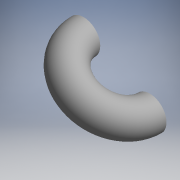
# Autodesk Inventor part: Half Off-Axis Donut Revolve Demo
Saved by Autodesk Inventor 2019 (Build 230136000, 136)
## iProperties
Part Number: Half Off-Axis Donut Revolve Demo
Material: Generic
Document SubType Name: Modeling
Designer: oriani
Appearance: Default
Author: oriani
Autodesk Inventor part; units mm, degrees
ref_plane "YZ Plane" through (0, 0, 0) normal (1, 0, 0) x (0, 1, 0)
ref_plane "XZ Plane" through (0, 0, 0) normal (0, 1, 0) x (-1, 0, 0)
ref_plane "XY Plane" through (0, 0, 0) normal (0, 0, 1) x (1, 0, 0)
sketch "Sketch1" plane through (0, 0, 0) normal (0, 0, 1) x (1, 0, 0)
  circle A0 centre (0, 25.4) radius 5.08
  line L0 (0, 0) -> (6.35, 12.7)
  dimension "d0" = 0
  constraints: 2 end point, 1 centre point
revolve "Revolution1" add sketch "Sketch1" angle 180 about axis through (0, 0, 0) along (0.4472, 0.8944, 0)
body "Solid1"
